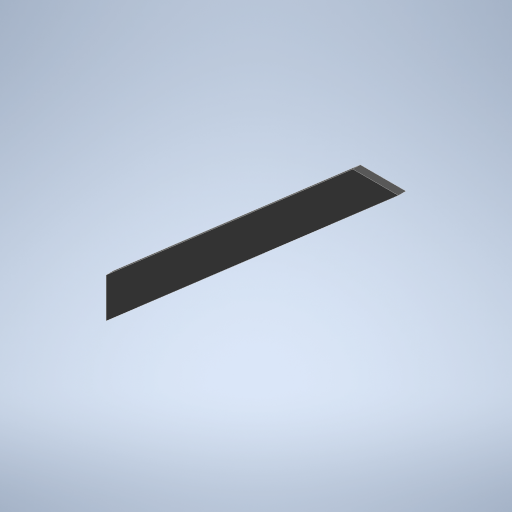
# Autodesk Inventor part: RP_Waist-Diagonal-material
Saved by Autodesk Inventor 2024.3 (Build 283343000, 343)
## iProperties
Created: 2025-05-22
Part Number: RP_Waist-Diagonal-material
Material: A5052
Document SubType Name: Modeling
Designer: 佐藤智貴
Density: 2.68 g/cm^3
Appearance: 一般
Mass: 117.02 g
Surface Area: 202.186 cm^2
Volume: 43.6643 cm^3
Author: 佐藤智貴
Autodesk Inventor part; units mm, degrees
ref_plane "YZ Plane" through (0, 0, 0) normal (1, 0, 0) x (0, 1, 0)
ref_plane "XZ Plane" through (0, 0, 0) normal (0, 1, 0) x (-1, 0, 0)
ref_plane "XY Plane" through (0, 0, 0) normal (0, 0, 1) x (1, 0, 0)
sketch "スケッチ1" plane through (0, 0, 0) normal (0, 0, 1) x (1, 0, 0)
  line L0 (0, 0) -> (195, 0)
  line L1 (195, 0) -> (195, 170)
  line L2 (195, 170) -> (0, 170)
  line L3 (0, 170) -> (0, 0)
  line L4 (0, 0) -> (195, 170)
  dimension "d0" = 195
  dimension "d1" = 170
  constraints: 10 end point, 2 parallel, 1 horizontal, 1 perpendicular
  measures "d0" distance of L1.end L2.end
  measures "d1" distance of L0.end L1.end
extrude "押し出し1" add sketch "スケッチ1" along normal blind 5 contours L3 L2 L4
sketch "スケッチ13" plane through (0, 0, 5) normal (0, 0, 1) x (1, 0, 0)
  line L0 (0, 0) -> (195, 170) projected
  line L1 (0, 0) -> (195, 170)
  line L2 (0, 0) -> (195, 170) projected
  line L3 (195, 170) -> (0, 170) projected
  line L4 (0, 170) -> (0, 0) projected
  line L5 (169.9396, 174.6857) -> (-13.756, 14.5408)
  line L6 (10, 160) -> (168.3118, 160)
  line L7 (168.3118, 160) -> (10, 21.9845)
  line L8 (10, 21.9845) -> (10, 160)
  point P0 (0, 26.5332)
  point P1 (164.5649, 170)
  point P2 (10, 35.2511)
  point P3 (153.0943, 160)
  dimension "d75" = 20
  dimension "d78" = 10
  constraints: 10 end point, 1 collinear, 1 parallel, 2 other
  measures "d75" distance between parallel lines of L0 L5
  measures "d78" distance between parallel lines of L3 L6
extrude "押し出し11" cut sketch "スケッチ13" against normal blind 10 contours L8 L6 L5
fillet "フィレット7" radius 5 3 edges at (10, 160, 2.5) (10, 35.2511, 2.5) (153.0943, 160, 2.5)
sketch "スケッチ14" plane through (0, 0, 5) normal (0, 0, 1) x (1, 0, 0)
  line L0 (15, 160) -> (139.7502, 160) projected
  arc A0 (143.0359, 151.2311) -> (139.7502, 160) centre (139.7502, 155) ccw projected
  line L1 (143.0359, 151.2311) -> (18.2857, 42.4746) projected
  arc A1 (10, 46.2434) -> (18.2857, 42.4746) centre (15, 46.2434) ccw projected
  line L2 (10, 46.2434) -> (10, 155) projected
  arc A2 (15, 160) -> (10, 155) centre (15, 155) ccw projected
  line L3 (0, 0) -> (195, 170) projected
  line L4 (195, 170) -> (0, 170) projected
  line L5 (0, 170) -> (0, 0) projected
  line L6 (164.5649, 170) -> (-7.7035, 19.8173)
  point P0 (143.0359, 151.2311)
  point P1 (0, 26.5332)
  point P2 (18.2857, 42.4746)
  dimension "d80" = 20
  constraints: 3 point on line, 2 end point
  measures "d80" distance between parallel lines of L3 L6
extrude "押し出し12" cut sketch "スケッチ14" against normal blind 10 contours A2 L2 A1 L6 L5 L4 A0 L0
